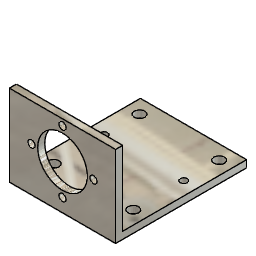
chapinhas (Autodesk Fusion 360 design; units mm, degrees)
Autodesk Fusion 360 part; units mm, degrees
sketch "Sketch1" plane through (0, 0, 0) normal (0, 0, 1) x (1, 0, 0)
  circle A0 centre (0, 0) radius 14
  circle A1 centre (17.5, 0) radius 2
  circle A2 centre (0, 17.5) radius 2
  circle A3 centre (-17.5, 0) radius 2
  circle A4 centre (0, -17.5) radius 2
  line L0 (30, -21) -> (-30, -21)
  line L1 (-30, -21) -> (-30, 21)
  line L2 (-30, 21) -> (30, 21)
  line L3 (30, 21) -> (30, -21)
  line L4 (-30, -21) -> (30, -21)
  line L5 (30, -21) -> (30, -25)
  line L6 (30, -25) -> (-30, -25)
  line L7 (-30, -25) -> (-30, -21)
  dimension "d2" = 28
  dimension "d4" = 4
  dimension "d6" = 360
  dimension "d7" = 60
  dimension "d8" = 42
  dimension "d9" = 60
  dimension "d10" = 4
  constraint horizontal L0
  constraint perpendicular L0 L1
  constraint parallel L0 L2
  constraint parallel L1 L3
  constraint coincident A0.centre origin
  constraint horizontal L4
  constraint vertical L5
  constraint horizontal L6
  constraint vertical L7
  measures "d2" diameter of A0
  measures "d4" diameter of A1
  measures "d4" distance of L0.end L6.end
extrude "Extrude1" add sketch "Sketch1" along normal blind 4
extrude "Extrude2" add sketch "Sketch1" against normal blind 70 contours L0 L4 L5 L6 L7
sketch "Sketch2" plane through (0, -25, 0) normal (0, -1, 0) x (1, 0, 0)
  line L0 (30, -70) -> (30, 4)
  line L1 (30, 4) -> (-30, 4)
  line L2 (-30, 4) -> (-30, -70)
  line L3 (-30, -70) -> (30, -70)
  circle A0 centre (-22.5, -13.5) radius 3
  circle A1 centre (-22.5, -42) radius 2
  circle A2 centre (-22.5, -62) radius 3
  circle A3 centre (22.5, -42) radius 2
  circle A4 centre (22.5, -62) radius 3
  circle A5 centre (22.5, -13.5) radius 3
  dimension "d24" = 6
  dimension "d25" = 4
  dimension "d26" = 6
  measures "d24" diameter of A0
  measures "d4" diameter of A1
  measures "d26" diameter of A2
extrude "Extrude3" cut sketch "Sketch2" against normal blind 10 contours A0 | A1 | A2 | A3 | A4 | A5
equation "d11 = d10"
